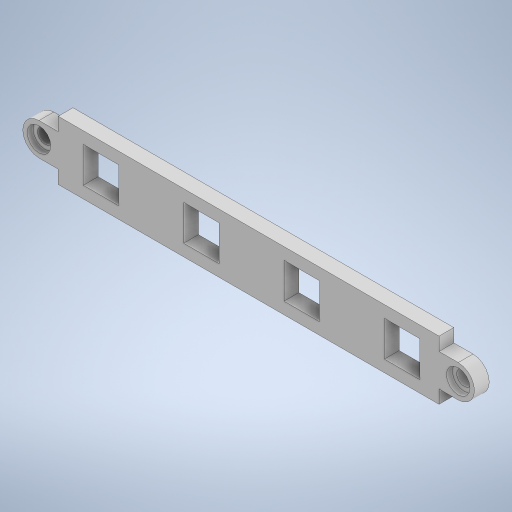
# Autodesk Inventor part: 네오픽셀 홀더
Saved by Autodesk Inventor 2023 (Build 270158000, 158)
## iProperties
Created: 2022-11-10
Part Number: 네오픽셀 홀더
Material: 일반
Document SubType Name: Modeling
Designer: user
Density: 1 g/cm^3
Appearance: 기본값
Author: user
Autodesk Inventor part; units mm, degrees
ref_plane "YZ Plane" through (0, 0, 0) normal (1, 0, 0) x (0, 1, 0)
ref_plane "XZ Plane" through (0, 0, 0) normal (0, 1, 0) x (-1, 0, 0)
ref_plane "XY Plane" through (0, 0, 0) normal (0, 0, 1) x (1, 0, 0)
sketch "스케치1" plane through (0, 0, 0) normal (0, 0, 1) x (1, 0, 0)
  line L0 (-32.25, 5) -> (32.25, 5)
  line L1 (32.25, 5) -> (32.25, -5)
  line L2 (32.25, -5) -> (-32.25, -5)
  line L3 (-32.25, -5) -> (-32.25, 5)
  line L4 (-32.25, 5) -> (32.25, -5) construction
  line L5 (32.25, 5) -> (-32.25, -5) construction
  circle A0 centre (-35.5, 0) radius 2.75
  circle A1 centre (-35.5, 0) radius 1.25
  line L6 (0, 0) -> (0, 3.25)
  circle A2 centre (35.5, 0) radius 2.75
  circle A3 centre (35.5, 0) radius 1.25
  line L7 (-35.5, 2.75) -> (-32.25, 2.75)
  line L8 (-35.5, -2.75) -> (-32.25, -2.75)
  line L9 (35.5, 2.75) -> (32.25, 2.75)
  line L10 (35.5, -2.75) -> (32.25, -2.75)
  dimension "d0" = 64.5
  dimension "d1" = 10
  dimension "d2" = 5.5
  dimension "d3" = 2.5
  dimension "d4" = 71
  constraints: 22 end point, 5 perpendicular, 4 centre point, 4 point on circle, 4 point on line, 2 coincident, 2 midpoint, 2 parallel, 2 symmetric about line, 2 tangent, 1 horizontal, 1 horizontal alignment, 1 vertical, 2 other
  measures "d0" distance of L1.end L2.end
  measures "d1" distance of L0.end L1.end
  measures "d2" diameter of A0
  measures "d3" diameter of A1
  measures "d4" distance of A2.centre A0.centre
extrude "돌출1" add sketch "스케치1" against normal blind 2.5
sketch "스케치2" plane through (0, 0, 0) normal (0, 0, 1) x (1, 0, 0)
  circle A0 centre (-35.5, 0) radius 1.25 projected
  circle A1 centre (-35.5, 0) radius 2
  circle A2 centre (35.5, 0) radius 1.25 projected
  circle A3 centre (35.5, 0) radius 2
  point P0 (0, 0)
  dimension "d7" = 4
  dimension "d8" = 4
  constraints: 2 centre point, 2 coincident
  measures "d7" diameter of A1
  measures "d8" diameter of A3
extrude "돌출2" cut sketch "스케치2" against normal blind 1 contours A0 | A1 | A2 | A3
sketch "스케치3" plane through (0, 0, 0) normal (0, 0, 1) x (1, 0, 0)
  line L0 (-28, 3) -> (-22, 3)
  line L1 (-22, 3) -> (-22, -3)
  line L2 (-22, -3) -> (-28, -3)
  line L3 (-28, -3) -> (-28, 3)
  line L4 (-28, 3) -> (-22, -3) construction
  line L5 (-22, 3) -> (-28, -3) construction
  line L6 (-11, 3) -> (-5, 3)
  line L7 (-5, 3) -> (-5, -3)
  line L8 (-5, -3) -> (-11, -3)
  line L9 (-11, -3) -> (-11, 3)
  line L10 (-11, 3) -> (-5, -3) construction
  line L11 (-5, 3) -> (-11, -3) construction
  line L12 (6, 3) -> (12, 3)
  line L13 (12, 3) -> (12, -3)
  line L14 (12, -3) -> (6, -3)
  line L15 (6, -3) -> (6, 3)
  line L16 (6, 3) -> (12, -3) construction
  line L17 (12, 3) -> (6, -3) construction
  line L18 (23, 3) -> (29, 3)
  line L19 (29, 3) -> (29, -3)
  line L20 (29, -3) -> (23, -3)
  line L21 (23, -3) -> (23, 3)
  line L22 (23, 3) -> (29, -3) construction
  line L23 (29, 3) -> (23, -3) construction
  point P0 (0, 0)
  point P1 (-25, 0)
  point P2 (-8, 0)
  point P3 (9, 0)
  point P4 (26, 0)
  dimension "d11" = 6
  dimension "d12" = 6
  dimension "d13" = 25
  dimension "d16" = 17
  constraints: 48 end point, 2 horizontal, 2 midpoint, 2 parallel, 1 collinear, 1 horizontal alignment, 1 perpendicular, 32 other
  measures "d11" distance of L1.end L2.end
  measures "d12" distance of L0.end L1.end
  measures "d13" distance of point (0, 0) point (-25, 0)
  measures "d16" distance of L0.start L6.start
extrude "돌출3" cut sketch "스케치3" against normal up to surface (2.5 mm away)
